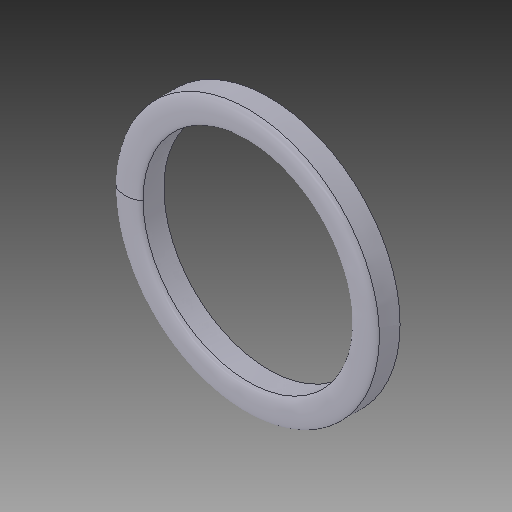
# Autodesk Inventor part: AxleWasher
Saved by Autodesk Inventor 2019 (Build 230136000, 136)
## iProperties
Created: 2020-12-09
Part Number: AxleWasher
Material: Stainless Steel AISI 440C, Welded
Document SubType Name: Modeling
Designer: Anass Hamdi
Density: 7.8 g/cm^3
Appearance: Weld - Stainless Steel
Author: Anass Hamdi
Autodesk Inventor part; units mm, degrees
ref_plane "YZ Plane" through (0, 0, 0) normal (1, 0, 0) x (0, 1, 0)
ref_plane "XZ Plane" through (0, 0, 0) normal (0, 1, 0) x (-1, 0, 0)
ref_plane "XY Plane" through (0, 0, 0) normal (0, 0, 1) x (1, 0, 0)
sketch "Sketch1" plane through (0, 0, 0) normal (0, 0, 1) x (1, 0, 0)
  circle A0 centre (0, 0) radius 4.05
  circle A1 centre (0, 0) radius 5.05
  dimension "d0" = 8.1
  dimension "d1" = 1
  constraints: 2 centre point, 2 coincident
  measures "d0" diameter of A0
  measures "d1" radial gap between concentric circles of A1 A0
extrude "Extrusion1" add sketch "Sketch1" along normal blind 0.8
sketch "Sketch2" plane through (0, 0, 0) normal (0, 1, 0) x (-1, 0, 0)
  line L0 (5.05, 0.8) -> (5.05, 0) projected
  line L1 (5.05, 0) -> (4.05, 0) projected
  line L2 (4.05, 0) -> (4.05, 0.8) projected
  line L3 (4.05, 0.8) -> (5.05, 0.8) projected
  line L4 (-5.05, 0) -> (-5.05, 0.8) projected
  line L5 (-5.05, 0.8) -> (-4.05, 0.8) projected
  line L6 (-4.05, 0.8) -> (-4.05, 0) projected
  line L7 (-4.05, 0) -> (-5.05, 0) projected
  line L8 (4.55, 0.8) -> (4.55, 1) construction
  ellipse E0 centre (4.55, 0.8) end of major axis (5.05, 0.8) minor radius 0.2 (5.05, 0.8) -> (4.05, 0.8) ccw
  line L9 (5.05, 0) -> (5.05, 0.8) projected
  line L10 (5.05, 0.8) -> (4.05, 0.8)
  line L11 (0, -0.2) -> (0, 1.2) projected
  point P0 (0, 0)
  dimension "d4" = 0.2
  constraints: 4 end point, 2 vertical, 1 coincident, 1 collinear, 1 midpoint, 6 other
  measures "d4" distance of L8.start L8.end
revolve "Revolution1" add sketch "Sketch2" angle 360 about axis through (0, 0, -10) along (0, 0, 1) contours L3 E0
body "Solid1"
